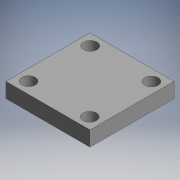
# Autodesk Inventor part: Part6
Saved by Autodesk Inventor 2016 (Build 200138000, 138)
## iProperties
Created: 2018-01-24
Part Number: Part6
Material: Generic
Document SubType Name: Modeling
Designer: student
Density: 1 g/cm^3
Appearance: Default
Author: student
Autodesk Inventor part; units mm, degrees
ref_plane "YZ Plane" through (0, 0, 0) normal (1, 0, 0) x (0, 1, 0)
ref_plane "XZ Plane" through (0, 0, 0) normal (0, 1, 0) x (-1, 0, 0)
ref_plane "XY Plane" through (0, 0, 0) normal (0, 0, 1) x (1, 0, 0)
sketch "Sketch1" plane through (0, 0, 0) normal (0, 1, 0) x (-1, 0, 0)
  circle A0 centre (-94.6824, 281.0189) radius 1.4224
  circle A1 centre (-94.7479, 264.89) radius 1.4224
  circle A2 centre (-80.524, 264.8323) radius 1.4224
  circle A3 centre (-80.4585, 280.9611) radius 1.4224
  line L0 (-96.4532, 263.3256) -> (-77.4032, 263.3256) construction
  line L1 (-96.4532, 282.4506) -> (-96.4532, 263.4006) construction
  line L2 (-78.7132, 281.8156) -> (-96.4932, 281.8156)
  line L3 (-96.4932, 281.8156) -> (-96.4932, 264.0356)
  line L4 (-96.4932, 264.0356) -> (-78.7132, 264.0356)
  line L5 (-78.7132, 264.0356) -> (-78.7132, 281.8156)
  line L6 (-78.7132, 281.8156) -> (-96.4932, 264.0356) construction
  line L7 (-96.4932, 281.8156) -> (-78.7132, 264.0356) construction
  circle A4 centre (-87.6032, 272.9256) radius 2.5
  point P0 (0, 0)
extrude "Extrusion1" add sketch "Sketch1" along normal blind 3.175 contours A0 L2 A3 L5 L4 A2 A1 L3
body "Solid1"
